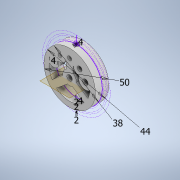
# Autodesk Inventor part: gimbal_inner_ring
Saved by Autodesk Inventor 2021 (Build 250183000, 183)
## iProperties
Created: 2021-06-14
Part Number: gimbal_inner_ring
Material: Generic
Document SubType Name: Modeling
Designer: Charlie
Density: 1 g/cm^3
Appearance: Default
Author: Charlie
Autodesk Inventor part; units mm, degrees
ref_plane "YZ Plane" through (0, 0, 0) normal (1, 0, 0) x (0, 1, 0)
ref_plane "XZ Plane" through (0, 0, 0) normal (0, 1, 0) x (-1, 0, 0)
ref_plane "XY Plane" through (0, 0, 0) normal (0, 0, 1) x (1, 0, 0)
sketch "Sketch1" plane through (0, 0, 0) normal (0, 0, 1) x (1, 0, 0)
  circle A0 centre (0, 0) radius 25 construction
  circle A1 centre (0, 0) radius 23 construction
  circle A2 centre (0, 0) radius 22 construction
  circle A3 centre (0, 0) radius 20 construction
  circle A4 centre (0, 0) radius 19
  circle A5 centre (0, 0) radius 17 construction
  line L0 (0, 25) -> (0, -25) construction
  line L1 (-25, 0) -> (25, 0) construction
  line L2 (0, -25) -> (0, -21)
  line L3 (0, 21) -> (0, 25)
  circle A6 centre (0, -19) radius 2
  line L4 (0, -17) -> (0, -21)
  circle A7 centre (0, 19) radius 2
  line L5 (0, 17) -> (0, 21)
  circle A8 centre (0, 0) radius 15
  dimension "d11" = 4
  dimension "d0" = 50
  dimension "d1" = 2
  dimension "d2" = 44
  dimension "d3" = 2
  dimension "d4" = 38
  dimension "d5" = 2
  dimension "d10" = 4
  dimension "d17" = 4
  constraints: 12 end point, 9 point on circle, 8 centre point, 3 coincident, 3 point on line, 1 collinear, 1 perpendicular, 3 other
  measures "d0" diameter of A0
  measures "d1" radial gap between concentric circles of A0 A1
  measures "d2" diameter of A2
  measures "d3" radial gap between concentric circles of A2 A3
  measures "d4" diameter of A4
  measures "d5" radial gap between concentric circles of A4 A5
  measures "d10" diameter of A6
  measures "d17" radial gap between concentric circles of A4 A8
extrude "Extrusion1" add sketch "Sketch1" along normal mid plane 10 contours A4 A6 A7 | A7 L5 A4 | A4 L4 A6 | L5 A7 A4 | A4 A6 L4 picked at (0.3657, 18.345) picked at (0.3657, -18.345) picked at (-0.3657, 18.345) picked at (-0.3657, -18.345)
revolve "Revolution1" cut sketch "Sketch1" angle 360 about axis through (0, -17, 0) along (0, -1, 0) picked at (0.5115, -19.5967) picked at (0.3657, -18.345) contours A6 L4 A4 | A4 L4 A6
revolve "Revolution2" cut sketch "Sketch1" angle 360 about axis through (0, 17, 0) along (0, -1, 0) picked at (0.3657, 18.345) picked at (0.5115, 19.5967) contours A7 L5 A4 | A4 L5 A7
sketch "Sketch2" plane through (0, 0, 5) normal (0, 0, 1) x (1, 0, 0)
  circle A0 centre (0, 12.5) radius 1.5
  circle A1 centre (-7.1601, 10.6767) radius 1.25
  circle A2 centre (-11.9448, 4.8266) radius 1
  circle A3 centre (7.4584, 9.48) radius 1.75
  circle A4 centre (11.6824, 3.0695) radius 2
  circle A5 centre (0, 0) radius 15 projected
  circle A6 centre (-11.9448, 4.8266) radius 4
  circle A7 centre (-7.1601, 10.6767) radius 4.25
  circle A8 centre (0, 12.5) radius 4.5
  circle A9 centre (7.4584, 9.48) radius 4.75
  circle A10 centre (11.6824, 3.0695) radius 5
  line L0 (-15.9448, 4.8266) -> (-10.5345, 13.2605)
  line L1 (-10.5345, 13.2605) -> (0, 17)
  arc A11 (-1.9972, 18.8947) -> (1.9972, 18.8947) centre (0, 19) ccw projected
  line L2 (0, 17) -> (11.6824, 11.6526)
  line L3 (11.6824, 11.6526) -> (16.6824, 3.0695)
  arc A12 (-1.5291, -1.2891) -> (-1.9312, 0.52) centre (0, 0) ccw
  circle A13 centre (0, 0) radius 5
  line L4 (-11.0597, -12.5939) -> (1.6114, -1.9114)
  line L5 (1.6114, -1.9114) -> (1.2891, -1.5291)
  line L6 (-1.6114, 1.9114) -> (-14.2825, -8.7712)
  line L7 (-14.2825, -8.7712) -> (-11.0597, -12.5939)
  line L8 (-11.0597, -12.5939) -> (-1.6114, 1.9114) construction
  line L9 (1.6114, -1.9114) -> (-14.2825, -8.7712) construction
  line L10 (12.2509, -11.6059) -> (-1.4315, -2.0496)
  line L11 (-1.4315, -2.0496) -> (-1.1452, -1.6397)
  line L12 (1.4315, 2.0496) -> (15.1139, -7.5067)
  line L13 (15.1139, -7.5067) -> (12.2509, -11.6059)
  line L14 (12.2509, -11.6059) -> (1.4315, 2.0496) construction
  line L15 (-1.4315, -2.0496) -> (15.1139, -7.5067) construction
  line L16 (2.5, 0.52) -> (2.5, 9.48)
  line L17 (2.5, 9.48) -> (-2.5, 9.48)
  line L18 (-2.5, 9.48) -> (-2.5, 0.52)
  line L19 (-2.5, 0.52) -> (-1.9312, 0.52)
  line L20 (2.5, 0.52) -> (-2.5, 9.48) construction
  line L21 (2.5, 9.48) -> (-2.5, 0.52) construction
  line L22 (-1.2891, 1.5291) -> (-1.6114, 1.9114)
  arc A14 (-1.9312, 0.52) -> (-1.5291, -1.2891) centre (0, 0) ccw
  line L23 (1.6397, -1.1452) -> (13.6824, -9.5563)
  line L24 (1.1452, 1.6397) -> (1.4315, 2.0496)
  line L25 (1.9312, 0.52) -> (2.5, 0.52)
  line L26 (-1.5291, -1.2891) -> (-12.6711, -10.6826)
  line L27 (0, 2) -> (0, 9.48)
  point P0 (0, 15)
  point P1 (-15, 0)
  point P2 (-6.3355, -5.3413)
  point P3 (6.8412, -4.7782)
  point P4 (0, 5)
  point P5 (-14.8548, 2.0821)
  point P6 (-8.3591, 6.5993)
  point P7 (-3.1455, 9.282)
  point P8 (-2.5, 8.7583)
  point P9 (-2.5, 4.3301)
  point P10 (-4.922, -0.8797)
  point P11 (-12.9193, -7.6219)
  point P12 (-9.6964, -11.4446)
  point P13 (-1.6992, -4.7024)
  point P14 (2.1185, -4.529)
  point P15 (10.694, -10.5185)
  point P16 (13.557, -6.4193)
  point P17 (4.9815, -0.4299)
  point P18 (2.5, 4.3301)
  point P19 (2.5, 8.7583)
  point P20 (2.7403, 8.9306)
  point P21 (6.9749, 4.7547)
  point P22 (14.9843, -0.6851)
  dimension "d30" = 4
  dimension "d31" = 3
  dimension "d18" = 3
  dimension "d19" = 2.5
  dimension "d20" = 2
  dimension "d21" = 3.5
  dimension "d22" = 4
  dimension "d23" = 12.5
  dimension "d24" = 30
  dimension "d25" = 3
  dimension "d26" = 3
  dimension "d27" = 3
  dimension "d28" = 3
  dimension "d29" = 3
  dimension "d32" = 5
  dimension "d33" = 5
  dimension "d34" = 5
  constraints: 56 end point, 12 parallel, 6 centre point, 6 midpoint, 5 perpendicular, 5 point on circle, 1 coincident, 1 point on line, 1 vertical, 29 other
  measures "d18" diameter of A0
  measures "d19" diameter of A1
  measures "d20" diameter of A2
  measures "d21" diameter of A3
  measures "d22" diameter of A4
  measures "d23" distance of A0.centre A5.centre
  measures "d24" diameter of A5
  measures "d27" diameter of A0
  measures "d32" distance of L6.start L4.end
  measures "d33" distance of L10.end L12.start
  measures "d34" distance of L17.end L16.end
extrude "Extrusion2" add sketch "Sketch2" against normal blind 5 contours A5 A10 A9 | A10 A9 A5 | A9 A10 A8 A5 | A9 A10 | A5 L23 A13 L12 | A9 A8 A5 | A5 L10 A13 L23 | L12 L16 A13 | A13 L23 A12 L25 L16 L12 | A9 A8 | A8 L16 L17 L18 A7 A5 A9 | A13 L10 L4 L5 A12 L23 | L16 L25 A12 L24 L12 | L12 L24 A12 L27 A13 L16 | L16 A13 L27 A8 | A8 L27 L17 L16 | A8 A7 A5 | A5 L26 A13 L4 | A13 L4 L10 | L27 A13 L18 A8 | A8 L18 L17 L27 | A7 A8 A6 A5 | A7 A8 | A5 L6 A13 L26 | A13 L26 A12 L11 L10 L4 | L10 L11 A12 L5 L4 | L27 A12 L22 L6 L18 A13 | A7 A6 A5 | A13 L6 L18 L19 A14 L26 | L18 L6 A13 | A6 A7 A5 | A6 A7 | L6 L22 A12 L19 L18
sketch "Sketch3" plane through (0, 0, 5) normal (0, 0, -1) x (1, 0, 0)
  circle A0 centre (0, 0) radius 2 projected
  circle A1 centre (0, 0) radius 2
  circle A2 centre (0, 0) radius 4
  circle A3 centre (0, 0) radius 2 projected
  point P0 (0, 2)
  dimension "d37" = 2
  constraints: 2 centre point, 1 coincident, 1 vertical alignment, 1 other
  measures "d37" radial gap between concentric circles of A0 A2
extrude "Extrusion4" add sketch "Sketch3" along normal blind 15
ref_plane "Work Plane1" through (0, -2, 5) normal (0, 1, 0) x (-1, 0, 0)
sketch "Sketch4" plane through (0, -2, 5) normal (0, 1, 0) x (-1, 0, 0)
  circle A0 centre (0, -10) radius 1.25
  line L0 (14.8548, -5) -> (-15, -5) projected
  point P0 (0, -5)
  point P1 (-14.9843, -5)
  dimension "d42" = 2.5
  dimension "d45" = 5
  constraints: 1 centre point
  measures "d42" diameter of A0
  measures "d45" distance from line of A0.centre L0
extrude "Extrusion5" cut sketch "Sketch4" along normal mid plane 5
fillet "Fillet1" radius 1 1 edges at (-4, 0, -10)
body "Solid1"
